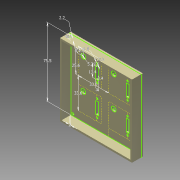
# Autodesk Inventor part: CameraBoardCover2
Saved by Autodesk Inventor 2015 (Build 190159000, 159)
## iProperties
Created: 2015-04-23
Part Number: CameraBoardCover2
Material: NylonD2W
Document SubType Name: Modeling
Designer: Akovo_000
Density: 1.13 g/cm^3
Appearance: Nylon 6
Mass: 23.2806 g
Surface Area: 217.65 cm^2
Volume: 20.6023 cm^3
Author: Akovo_000
Autodesk Inventor part; units mm, degrees
ref_plane "YZ Plane" through (0, 0, 0) normal (1, 0, 0) x (0, 1, 0)
ref_plane "XZ Plane" through (0, 0, 0) normal (0, 1, 0) x (-1, 0, 0)
ref_plane "XY Plane" through (0, 0, 0) normal (0, 0, 1) x (1, 0, 0)
sketch "Sketch1" plane through (0, 0, 0) normal (0, 1, 0) x (-1, 0, 0)
  line L0 (11.073, 25.2979) -> (-64.427, 25.2979)
  line L1 (-64.427, 25.2979) -> (-64.427, -50.2021)
  line L2 (-64.427, -50.2021) -> (11.073, -50.2021)
  line L3 (11.073, -50.2021) -> (11.073, 25.2979)
  circle A0 centre (8.873, 23.0979) radius 1.1
  circle A1 centre (-62.227, 23.0979) radius 1.1
  circle A2 centre (-62.227, -48.0021) radius 1.1
  circle A3 centre (8.873, -48.0021) radius 1.1
  line L4 (8.873, 23.0979) -> (11.073, 23.0979) construction
  line L5 (8.873, 23.0979) -> (8.873, 25.2979) construction
  line L6 (-62.227, 25.2979) -> (-62.227, 23.0979) construction
  line L7 (-62.227, 23.0979) -> (-64.427, 23.0979) construction
  line L8 (8.873, -48.0021) -> (11.073, -48.0021) construction
  line L9 (8.873, -48.0021) -> (8.873, -50.2021) construction
  line L10 (-62.227, -48.0021) -> (-64.427, -48.0021) construction
  line L11 (-62.227, -48.0021) -> (-62.227, -50.2021) construction
  line L12 (2.923, 17.1479) -> (-22.677, 17.1479) construction
  line L13 (-22.677, 17.1479) -> (-22.677, -8.4521) construction
  line L14 (-22.677, -8.4521) -> (2.923, -8.4521) construction
  line L15 (2.923, -8.4521) -> (2.923, 17.1479) construction
  circle A4 centre (-2.577, 12.7479) radius 2.6
  line L16 (13.073, 27.2979) -> (-66.427, 27.2979)
  line L17 (-66.427, 27.2979) -> (-66.427, -52.2021)
  line L18 (-66.427, -52.2021) -> (13.073, -52.2021)
  line L19 (13.073, -52.2021) -> (13.073, 27.2979)
  line L20 (-26.677, 25.2979) -> (-26.677, 27.2979) construction
  line L21 (13.073, -12.4521) -> (11.073, -12.4521) construction
  line L22 (-16.277, 11.0479) -> (-19.277, 11.0479)
  line L23 (-19.277, 11.0479) -> (-19.277, -2.3521)
  line L24 (-19.277, -2.3521) -> (-16.277, -2.3521)
  line L25 (-16.277, -2.3521) -> (-16.277, 11.0479)
  circle A5 centre (-17.777, -4.8521) radius 0.9
  circle A6 centre (-17.777, 13.5479) radius 0.9
  line L26 (-17.777, -4.8521) -> (-17.777, -2.3521) construction
  line L27 (-17.777, 13.5479) -> (-17.777, 11.0479) construction
  line L28 (-17.777, 13.5479) -> (-17.777, 17.1479) construction
  line L29 (-17.777, -4.8521) -> (-17.777, -8.4521) construction
  line L30 (6.873, 25.2979) -> (6.873, 21.0979) construction
  line L31 (6.873, 21.0979) -> (11.073, 21.0979) construction
  line L32 (2.923, -16.4521) -> (-22.677, -16.4521) construction
  line L33 (-22.677, -16.4521) -> (-22.677, -42.0521) construction
  line L34 (-22.677, -42.0521) -> (2.923, -42.0521) construction
  line L35 (2.923, -42.0521) -> (2.923, -16.4521) construction
  circle A7 centre (-2.577, -20.8521) radius 2.6
  line L36 (-16.277, -22.5521) -> (-19.277, -22.5521)
  line L37 (-19.277, -22.5521) -> (-19.277, -35.9521)
  line L38 (-19.277, -35.9521) -> (-16.277, -35.9521)
  line L39 (-16.277, -35.9521) -> (-16.277, -22.5521)
  circle A8 centre (-17.777, -38.4521) radius 0.9
  circle A9 centre (-17.777, -20.0521) radius 0.9
  line L40 (-17.777, -38.4521) -> (-17.777, -35.9521) construction
  line L41 (-17.777, -20.0521) -> (-17.777, -22.5521) construction
  line L42 (-17.777, -20.0521) -> (-17.777, -16.4521) construction
  line L43 (-17.777, -38.4521) -> (-17.777, -42.0521) construction
  line L44 (-30.677, 17.1479) -> (-56.277, 17.1479) construction
  line L45 (-56.277, 17.1479) -> (-56.277, -8.4521) construction
  line L46 (-56.277, -8.4521) -> (-30.677, -8.4521) construction
  line L47 (-30.677, -8.4521) -> (-30.677, 17.1479) construction
  circle A10 centre (-36.177, 12.7479) radius 2.6
  line L48 (-49.877, 11.0479) -> (-52.877, 11.0479)
  line L49 (-52.877, 11.0479) -> (-52.877, -2.3521)
  line L50 (-52.877, -2.3521) -> (-49.877, -2.3521)
  line L51 (-49.877, -2.3521) -> (-49.877, 11.0479)
  circle A11 centre (-51.377, -4.8521) radius 0.9
  circle A12 centre (-51.377, 13.5479) radius 0.9
  line L52 (-51.377, -4.8521) -> (-51.377, -2.3521) construction
  line L53 (-51.377, 13.5479) -> (-51.377, 11.0479) construction
  line L54 (-51.377, 13.5479) -> (-51.377, 17.1479) construction
  line L55 (-51.377, -4.8521) -> (-51.377, -8.4521) construction
  line L56 (-30.677, -16.4521) -> (-56.277, -16.4521) construction
  line L57 (-56.277, -16.4521) -> (-56.277, -42.0521) construction
  line L58 (-56.277, -42.0521) -> (-30.677, -42.0521) construction
  line L59 (-30.677, -42.0521) -> (-30.677, -16.4521) construction
  circle A13 centre (-36.177, -20.8521) radius 2.6
  line L60 (-49.877, -22.5521) -> (-52.877, -22.5521)
  line L61 (-52.877, -22.5521) -> (-52.877, -35.9521)
  line L62 (-52.877, -35.9521) -> (-49.877, -35.9521)
  line L63 (-49.877, -35.9521) -> (-49.877, -22.5521)
  circle A14 centre (-51.377, -38.4521) radius 0.9
  circle A15 centre (-51.377, -20.0521) radius 0.9
  line L64 (-51.377, -38.4521) -> (-51.377, -35.9521) construction
  line L65 (-51.377, -20.0521) -> (-51.377, -22.5521) construction
  line L66 (-51.377, -20.0521) -> (-51.377, -16.4521) construction
  line L67 (-51.377, -38.4521) -> (-51.377, -42.0521) construction
  line L68 (-56.277, 17.1479) -> (-64.427, 17.1479) construction
  line L69 (2.923, 17.1479) -> (11.073, 17.1479) construction
  line L70 (-30.677, 17.1479) -> (-30.677, 25.2979) construction
  line L71 (-30.677, -42.0521) -> (-30.677, -50.2021) construction
  dimension "d48" = 75.5
  dimension "d49" = 2.2
  dimension "d51" = 2.2
  dimension "d54" = 5.2
  dimension "d55" = 4.4
  dimension "d56" = 5.5
  dimension "d57" = 2
  dimension "d58" = 1.8
  dimension "d59" = 2.5
  dimension "d60" = 13.4
  dimension "d61" = 3
  dimension "d62" = 3.4
  dimension "d64" = 4.2
  dimension "d67" = 33.6
  dimension "d70" = 33.6
  dimension "d73" = 25.6
  dimension "d74" = 25.6
  constraints: 144 end point, 28 point on line, 19 perpendicular, 16 centre point, 14 equal length, 8 parallel, 6 horizontal, 6 midpoint, 4 equal radius, 2 vertical, 90 other
  measures "d48" distance of L2.end L0.start
  measures "d49" diameter of A0
  measures "d51" distance of L0.start L4.end
  measures "d54" diameter of A4
  measures "d55" distance from line of L12 A4.centre
  measures "d56" distance from line of L15 A4.centre
  measures "d57" horizontal distance of L2.end L18.end
  measures "d58" diameter of A6
  measures "d59" distance of L27.start L27.end
  measures "d60" distance between parallel lines of L24 L22
  measures "d61" distance between parallel lines of L23 L25
  measures "d62" distance between parallel lines of L13 L23
  measures "d64" distance of L0.start L31.end
  measures "d67" distance of L14.end L35.start
  measures "d70" distance of L14.end L47.start
  measures "d73" distance of L14.end L12.start
  measures "d74" distance of L12.end L12.start
extrude "Edges" add sketch "Sketch1" against normal blind 10 contours L19 L18 L17 L16
extrude "Surface" add sketch "Sketch1" along normal blind 2 contours L3 L2 L1 L0 | L19 L18 L17 L16
body "Solid1"
